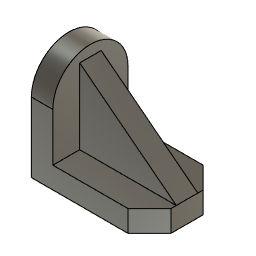
A1 (Autodesk Fusion 360 design; units mm, degrees)
Autodesk Fusion 360 part; units mm, degrees
sketch "Sketch1" plane through (0, 0, 0) normal (0, 0, 1) x (1, 0, 0)
  line L0 (54, -42) -> (0, -42)
  line L1 (0, -42) -> (0, 0)
  line L2 (66, -42) -> (54, -42) construction
  line L3 (54, -42) -> (54, -30) construction
  line L4 (54, -30) -> (66, -30) construction
  line L5 (54, -42) -> (66, -30)
  line L6 (54, 0) -> (54, -12) construction
  line L7 (54, -12) -> (66, -12) construction
  line L8 (66, -12) -> (54, 0)
  line L9 (66, -30) -> (66, -12)
  line L10 (66, 0) -> (66, -12) construction
  line L11 (66, -30) -> (66, -42) construction
  line L12 (54, 0) -> (0, 0)
  line L13 (54, 0) -> (66, 0) construction
  line L14 (0, -42) -> (12, -42)
  line L15 (12, -42) -> (12, 0)
  line L16 (12, 0) -> (0, 0)
  line L17 (0, 0) -> (0, -42)
  line L18 (12, -21) -> (12, -15)
  line L19 (12, -15) -> (66, -15)
  line L20 (12, -21) -> (12, -27)
  line L21 (12, -27) -> (66, -27)
  line L22 (12, -21) -> (66, -21)
  dimension "d1" = 42
  dimension "d3" = 12
  dimension "d4" = 12
  dimension "d7" = 54
  dimension "d8" = 12
  dimension "d10" = 12
  dimension "d11" = 6
  dimension "d12" = 6
  dimension "d13" = 66
  dimension "d14" = 42
  constraint horizontal L0
  constraint vertical L1
  constraint coincident L1.end L12.end
  constraint horizontal L2
  constraint vertical L3
  constraint horizontal L4
  constraint vertical L6
  constraint horizontal L7
  constraint perpendicular L7 L9
  constraint perpendicular L7 L10
  constraint perpendicular L2 L11
  constraint perpendicular L1 L12
  constraint perpendicular L10 L13
  constraint horizontal L14
  constraint vertical L15
  constraint horizontal L16
  constraint vertical L17
  constraint coincident L12 L15.end
  constraint midpoint L15 L18.start
  constraint coincident L9 L19.end
  constraint perpendicular L9 L19
  constraint coincident L9 L21.end
  constraint perpendicular L9 L21
  constraint midpoint L9 L22.end
  measures "d1" distance of L1.end L0.end
  measures "d3" distance of L2.start L4.end
  measures "d4" distance of L2.start L0.start
  measures "d7" distance of L0.end L0.start
  measures "d8" distance of L0.end L14.end
  measures "d10" distance of L7.end L10.start
  measures "d11" distance of L18.start L18.end
  measures "d12" distance of L18.start L20.end
  measures "d13" distance of L1.end L10.start
  measures "d14" distance of L2.start L10.start L1.end
extrude "Extrude1" add sketch "Sketch1" along normal blind 60 contours L0 L1 L12 L14 L15 L16 L17 L18 L20
extrude "Extrude2" add sketch "Sketch1" along normal blind 12 contours L0 L5 L9 L15 L21 | L9 L15 L20 L21 L22 | L9 L15 L18 L19 L22 | L8 L9 L12 L15 L19
fillet "Fillet1" radius 21 1 edges at (6, -42, 60)
fillet "Fillet2" radius 21 1 edges at (6, 0, 60)
ref_plane "WorkPlane1" through (27, -21, 19.5) normal (0, 1, 0) x (-1, 0, 0)
sketch "Sketch3" plane through (27, -21, 19.5) normal (0, 1, 0) x (1, 0, 0)
  line L0 (-15, -34.5) -> (39, 7.5)
  line L1 (39, 7.5) -> (-15, 7.5)
  line L2 (-15, 7.5) -> (-15, -34.5)
  line L3 (-15, 7.5) -> (27, 7.5)
  line L4 (-15, 7.5) -> (-15, -19.5)
  point P0 (39, 7.5)
  dimension "d21" = 42
  constraint horizontal L1
  constraint perpendicular L1 L2
  constraint collinear L1 L3
  constraint collinear L2 L4
  constraint coincident P0 L0.end
  measures "d21" distance of L0.start L1.end
extrude "Extrude3" add sketch "Sketch3" along normal blind 6 and the other way blind 6
